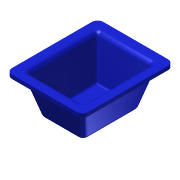
# Autodesk Inventor part: Rail car yellow
Saved by Autodesk Inventor 2015 (Build 190159000, 159)
## iProperties
Created: 2015-03-08
Part Number: Rail car yellow
Material: Generic
Document SubType Name: Modeling
Designer: Vukica
Density: 1 g/cm^3
Appearance: Blue - Wall Paint - Glossy
Author: Vukica
Autodesk Inventor part; units mm, degrees
ref_plane "YZ Plane" through (0, 0, 0) normal (1, 0, 0) x (0, 1, 0)
ref_plane "XZ Plane" through (0, 0, 0) normal (0, 1, 0) x (-1, 0, 0)
ref_plane "XY Plane" through (0, 0, 0) normal (0, 0, 1) x (1, 0, 0)
sketch "Sketch1" plane through (0, 0, 0) normal (0, 1, 0) x (-1, 0, 0)
  line L0 (0, 0) -> (177.8, 0)
  line L1 (177.8, 0) -> (177.8, -260.35)
  line L2 (177.8, -260.35) -> (0, -260.35)
  line L3 (0, -260.35) -> (0, 0)
  dimension "d0" = 260.35
  dimension "d1" = 177.8
  constraints: 8 end point, 2 parallel, 1 horizontal, 1 perpendicular
  measures "d0" distance of L0.end L1.end
  measures "d1" distance of L1.end L2.end
extrude "Extrusion1" add sketch "Sketch1" along normal blind 133.35
draft "FaceDraft1" angle -15 pull direction (0, 1, 0) faces at (-59.2667, 44.45, 0) (0, 44.45, -173.5667) (-118.5333, 44.45, -260.35) (-177.8, 88.9, -86.7833) fixed edges at (-88.9, 133.35, 0) (0, 133.35, -130.175) (-88.9, 133.35, -260.35) (-177.8, 0, -130.175)
fillet "Fillet1" radius 19.05 8 edges at (-17.8655, 66.675, -17.8655) (-195.6655, 66.675, -17.8655) (-17.8655, 66.675, -242.4845) (-195.6655, 66.675, -242.4845) (-177.8, 0, -130.175) (-106.7655, 0, -35.731) (-35.731, 0, -130.175) (-106.7655, 0, -224.619)
shell "Shell2" thickness 12.7 removed faces 1 at (-142.354, 133.35, -167.433)
sketch "Sketch2" plane through (0, 133.35, 0) normal (0, 1, 0) x (1, 0, 0)
  ellipse E0 centre (-19.722, 19.722) end of major axis (-14.9203, 14.9203) minor radius 6.35 (-19.2816, 13.148) -> (-13.148, 19.2816) ccw projected
  line L0 (-19.2816, 13.148) -> (-194.2494, 13.148) projected
  line L1 (-13.148, 241.0684) -> (-13.148, 19.2816) projected
  line L2 (-200.383, 19.2816) -> (-200.383, 241.0684) projected
  ellipse E1 centre (-193.809, 19.722) end of major axis (-198.6107, 14.9203) minor radius 6.35 (-200.383, 19.2816) -> (-194.2494, 13.148) ccw projected
  ellipse E2 centre (-193.809, 240.628) end of major axis (-198.6107, 245.4297) minor radius 6.35 (-194.2494, 247.202) -> (-200.383, 241.0684) ccw projected
  line L3 (-194.2494, 247.202) -> (-19.2816, 247.202) projected
  ellipse E3 centre (-19.722, 240.628) end of major axis (-14.9203, 245.4297) minor radius 6.35 (-13.148, 241.0684) -> (-19.2816, 247.202) ccw projected
  line L4 (20.2345, -22.225) -> (-233.7655, -22.225)
  line L5 (-233.7655, -22.225) -> (-233.7655, 282.575)
  line L6 (-233.7655, 282.575) -> (20.2345, 282.575)
  line L7 (20.2345, 282.575) -> (20.2345, -22.225)
  line L8 (0, 18.4009) -> (0, 241.9491) projected
  line L9 (-213.531, 241.9491) -> (-213.531, 18.4009) projected
  line L10 (-195.1301, 0) -> (-18.4009, 0) projected
  line L11 (-18.4009, 260.35) -> (-195.1301, 260.35) projected
  point P0 (0, 0)
  dimension "d17" = 254
  dimension "d18" = 304.8
  dimension "d19" = 213.531
  dimension "d20" = 20.2345
  dimension "d21" = 260.35
  dimension "d22" = 22.225
  constraints: 8 end point, 2 parallel, 1 horizontal, 1 perpendicular, 4 other
  measures "d17" distance between parallel lines of L7 L5
  measures "d18" distance of L4.end L5.end
  measures "d19" distance between parallel lines of L8 L9
  measures "d20" distance between parallel lines of L5 L9
  measures "d21" distance between parallel lines of L11 L10
  measures "d22" distance between parallel lines of L4 L10
extrude "Extrusion2" add sketch "Sketch2" against normal blind 12.7
fillet "Fillet2" radius 19.05 4 edges at (20.2345, 127, 22.225) (-233.7655, 127, -282.575) (20.2345, 127, -282.575) (-233.7655, 127, 22.225)
fillet "Fillet3" radius 19.05 8 edges at (-198.6107, 133.35, -14.9203) (-200.383, 133.35, -130.175) (-198.6107, 133.35, -245.4297) (-106.7655, 133.35, -247.202) (-14.9203, 133.35, -245.4297) (-13.148, 133.35, -130.175) (-14.9203, 133.35, -14.9203) (-106.7655, 133.35, -13.148)
equation "\"d20\" = -0.5 * d19 + 0.5 * d17"
equation "\"d22\" = -0.5 * d21 + 0.5 * d18"
body "Solid1"
